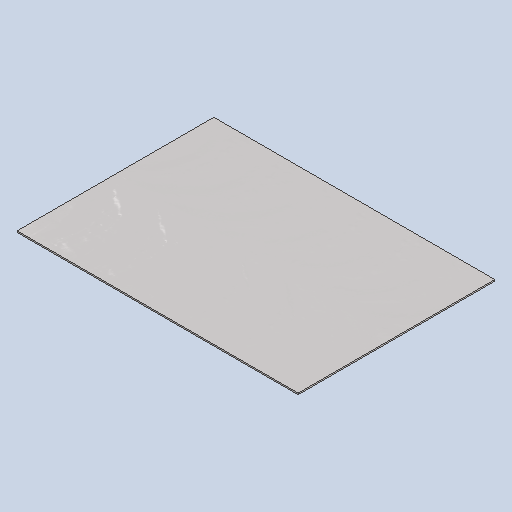
# Autodesk Inventor part: dach
Saved by Autodesk Inventor 2023 (Build 270158000, 158)
## iProperties
Created: 2023-07-07
Part Number: dach
Material: Stal miękka, spawana
Document SubType Name: Modeling
Designer: Kamil
Density: 7.85 g/cm^3
Appearance: Spawane — stal miękka
Author: Kamil
Autodesk Inventor part; units mm, degrees
ref_plane "YZ Plane" through (0, 0, 0) normal (1, 0, 0) x (0, 1, 0)
ref_plane "XZ Plane" through (0, 0, 0) normal (0, 1, 0) x (-1, 0, 0)
ref_plane "XY Plane" through (0, 0, 0) normal (0, 0, 1) x (1, 0, 0)
sketch "Szkic1" plane through (0, 0, 0) normal (0, 1, 0) x (-1, 0, 0)
  line L0 (0, 0) -> (-100, 0)
  line L1 (-100, 0) -> (-100, -70)
  line L2 (-100, -70) -> (0, -70)
  line L3 (0, -70) -> (0, 0)
  dimension "d0" = 100
  dimension "d1" = 70
  constraints: 8 end point, 2 parallel, 1 horizontal, 1 perpendicular
  measures "d0" distance of L2.end L1.end
  measures "d1" distance of L1.end L0.end
extrude "Wyciągnięcie proste1" add sketch "Szkic1" along normal blind 0.5
